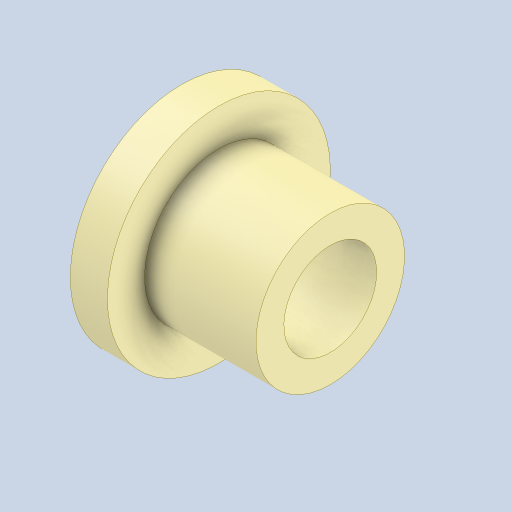
# Autodesk Inventor part: Nylon Slider
Saved by Autodesk Inventor 2024 (Build 280153000, 153)
## iProperties
Created: 2023-11-21
Part Number: Nylon Slider
Material: Nylon 6/6
Document SubType Name: Modeling
Designer: Greg
Density: 1.13 g/cm^3
Appearance: Nylon 6
Author: Greg
Autodesk Inventor part; units mm, degrees
ref_plane "YZ Plane" through (0, 0, 0) normal (1, 0, 0) x (0, 1, 0)
ref_plane "XZ Plane" through (0, 0, 0) normal (0, 1, 0) x (-1, 0, 0)
ref_plane "XY Plane" through (0, 0, 0) normal (0, 0, 1) x (1, 0, 0)
sketch "Sketch1" plane through (0, 0, 0) normal (0, 0, 1) x (1, 0, 0)
  line L0 (0, 0) -> (6.4727, 0) construction
  line L1 (0, 1.9844) -> (6.35, 1.9844)
  line L2 (6.35, 1.9844) -> (6.35, 3.175)
  line L3 (6.35, 3.175) -> (1.5875, 3.175)
  line L4 (1.5875, 3.175) -> (1.5875, 4.7625)
  line L5 (1.5875, 4.7625) -> (0, 4.7625)
  line L6 (0, 4.7625) -> (0, 1.9844)
  dimension "d1" = 4.7625
  dimension "d5" = 9.525
  dimension "d6" = 3.9688
  dimension "d7" = 6.35
  dimension "d8" = 6.35
  constraints: 14 end point, 5 perpendicular, 2 horizontal, 1 vertical alignment
  measures "d1" distance of L2.end L3.end
  measures "d5" diameter of L5 L0
  measures "d6" diameter of L1 L0
  measures "d7" diameter of L3 L0
  measures "d8" distance between parallel lines of L2 L6
revolve "Revolution1" add sketch "Sketch1" angle 360 about axis through (0, 0, 0) along (1, 0, 0)
body "Solid1"
